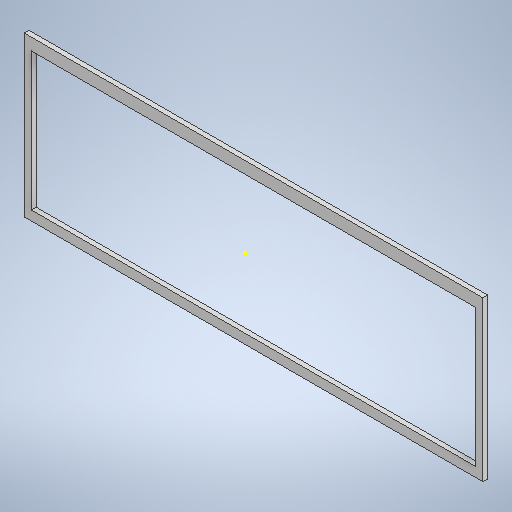
# Autodesk Inventor part: Front cover
Saved by Autodesk Inventor 2025.2 (Build 292293000, 293)
## iProperties
Created: 2025-04-05
Part Number: Front cover
Material: Generic
Document SubType Name: Modeling
Designer: pipep
Density: 1 g/cm^3
Appearance: Default
Author: pipep
Autodesk Inventor part; units mm, degrees
ref_plane "YZ Plane" through (0, 0, 0) normal (1, 0, 0) x (0, 1, 0)
ref_plane "XZ Plane" through (0, 0, 0) normal (0, 1, 0) x (-1, 0, 0)
ref_plane "XY Plane" through (0, 0, 0) normal (0, 0, 1) x (1, 0, 0)
sketch "Sketch1" plane through (0, 0, 0) normal (0, 0, 1) x (1, 0, 0)
  line L0 (0, 0) -> (92.58, 0)
  line L1 (92.58, 0) -> (92.58, 33.35)
  line L2 (92.58, 33.35) -> (-92.58, 33.35)
  line L3 (-92.58, 33.35) -> (-92.58, -33.35)
  line L4 (-92.58, -33.35) -> (92.58, -33.35)
  line L5 (92.58, -33.35) -> (92.58, 33.35)
  line L6 (-92.58, 33.35) -> (-89.58, 33.35)
  line L7 (-89.58, 33.35) -> (-89.58, 28.35)
  line L8 (92.58, -33.35) -> (89.58, -33.35)
  line L9 (89.58, -33.35) -> (89.58, -28.35)
  line L10 (-89.58, 28.35) -> (89.58, 28.35)
  line L11 (89.58, 28.35) -> (89.58, -28.35)
  line L12 (89.58, -28.35) -> (-89.58, -28.35)
  line L13 (-89.58, -28.35) -> (-89.58, 28.35)
  dimension "d0" = 92.58
  dimension "d1" = 33.35
  dimension "d2" = 185.16
  dimension "d3" = 66.7
  dimension "d4" = 3
  dimension "d5" = 5
  dimension "d6" = 3
  dimension "d7" = 5
  constraints: 28 end point, 4 parallel, 4 perpendicular, 3 horizontal, 2 point on line, 1 vertical
  measures "d0" distance of L0.start L0.end
  measures "d1" distance of L0.end L1.end
  measures "d2" distance of L4.end L3.end
  measures "d3" distance of L3.end L2.end
  measures "d4" distance of L2.end L6.end
  measures "d5" distance of L6.end L7.end
  measures "d6" distance of L4.end L8.end
  measures "d7" distance of L8.end L9.end
extrude "Extrusion1" add sketch "Sketch1" along normal blind 2 contours L11 L10 L7 L2 L1 L0 | L0 L5 L4 L9 L11 | L9 L4 L3 L2 L7 L13 L12
sketch "Sketch2" plane through (-89.58, -28.35, 0) normal (0, 1, 0) x (1, 0, 0)
  line L0 (179.16, -2) -> (0, -2) projected
  line L1 (0, 0) -> (179.16, 0)
  line L2 (179.16, 0) -> (179.16, -2)
  line L3 (179.16, -2) -> (0, -2)
  line L4 (0, -2) -> (0, 0)
  point P0 (89.58, 0)
  constraints: 8 end point, 2 parallel, 1 horizontal, 1 perpendicular
extrude "Extrusion2" cut sketch "Sketch2" against normal blind 1
sketch "Sketch3" plane through (0, 0, 2) normal (0, 0, 1) x (1, 0, 0)
  point P0 (0, 0)
sketch "Sketch4" plane through (0, 0, 2) normal (0, 0, 1) x (1, 0, 0)
  line L0 (92.58, -33.35) -> (92.58, 33.35) projected
  line L1 (92.58, 33.35) -> (99.58, 33.35)
  line L2 (99.58, 33.35) -> (99.58, -33.35)
  line L3 (99.58, -33.35) -> (92.58, -33.35)
  line L4 (89.58, 28.35) -> (89.58, -29.35) projected
  line L5 (89.58, -29.35) -> (96.58, -29.35)
  line L6 (96.58, -29.35) -> (96.58, 28.35)
  line L7 (96.58, 28.35) -> (89.58, 28.35)
  point P0 (0, 0)
  point P1 (92.58, 28.35)
  point P2 (92.58, -29.35)
  dimension "d12" = 7
  dimension "d13" = 90
  dimension "d14" = 7
  dimension "d15" = 90
  constraints: 12 end point, 3 perpendicular, 1 horizontal
  measures "d12" distance of L0.end L1.end
  measures "d13" angle of L1 L2
  measures "d14" distance of L4.end L5.end
  measures "d15" angle of L6 L5
extrude "Extrusion3" add sketch "Sketch4" against normal blind 2 contours L0 L5 L6 L7 L1 L2 L3
sketch "Sketch5" plane through (0, 0, 2) normal (0, 0, 1) x (1, 0, 0)
  line L0 (-89.58, 28.35) -> (89.58, 28.35) projected
  line L1 (96.58, -29.35) -> (92.58, -29.35) projected
  line L2 (89.58, 28.35) -> (92.58, 28.35)
  line L3 (92.58, 28.35) -> (92.58, -29.35)
  line L4 (92.58, -29.35) -> (89.58, -29.35)
  line L5 (89.58, -29.35) -> (89.58, 28.35)
  point P0 (0, 0)
  constraints: 8 end point, 2 parallel, 1 horizontal, 1 perpendicular
extrude "Extrusion4" cut sketch "Sketch5" against normal blind 2
equation "\"d2\" = 2 * d0"
equation "\"d3\" = 2 * d1"
body "Solid1"
